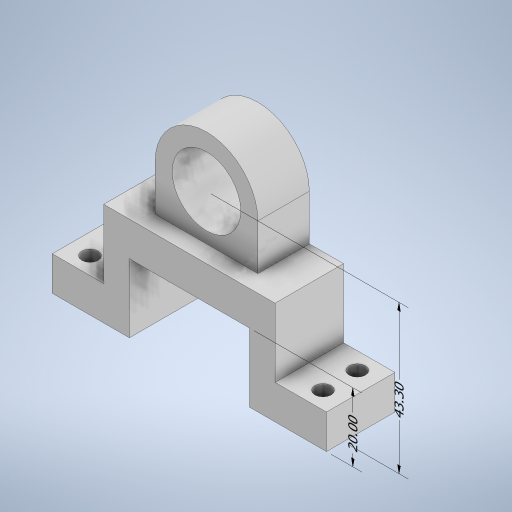
# Autodesk Inventor part: soporte_balineras
Saved by Autodesk Inventor 2023 (Build 270158000, 158)
## iProperties
Created: 2023-06-06
Part Number: soporte_balineras
Material: Genérico
Document SubType Name: Modeling
Designer: sergi
Density: 1 g/cm^3
Appearance: Valor por defecto
Author: sergi
Autodesk Inventor part; units mm, degrees
ref_plane "YZ Plane" through (0, 0, 0) normal (1, 0, 0) x (0, 1, 0)
ref_plane "XZ Plane" through (0, 0, 0) normal (0, 1, 0) x (-1, 0, 0)
ref_plane "XY Plane" through (0, 0, 0) normal (0, 0, 1) x (1, 0, 0)
sketch "Boceto1" plane through (0, 0, 0) normal (0, 0, 1) x (1, 0, 0)
  circle A0 centre (0, 23.4183) radius 10
  circle A1 centre (0, 23.4183) radius 15
  line L0 (-15, 23.4183) -> (-15, -2.7)
  line L1 (15, 23.4183) -> (15, -2.7)
  line L2 (-25, 0.1183) -> (25, 0.1183)
  line L3 (25, 0.1183) -> (25, 10.1183)
  line L4 (25, 10.1183) -> (-25, 10.1183)
  line L5 (-25, 10.1183) -> (-25, 0.1183)
  point P0 (0, 0)
  point P1 (0, 0.1183)
  point P2 (-15, 10.1183)
  point P3 (15, 10.1183)
  dimension "d0" = 20
  dimension "d1" = 30
  dimension "d2" = 50
  dimension "d11" = 10
  dimension "d23" = 23.3
  constraints: 12 end point, 2 centre point, 2 parallel, 2 point on circle, 2 vertical, 1 coincident, 1 horizontal, 1 midpoint, 1 perpendicular, 1 vertical alignment
  measures "d0" diameter of A0
  measures "d1" diameter of A1
  measures "d2" distance of L2.start L2.end
  measures "d11" distance of L2.end L3.end
  measures "d23" distance from line of L2 A0.centre
extrude "Extrusión1" add sketch "Boceto1" along normal blind 20 contours L4 L1 L2 L0 A1 | A1 L4 | L4 L3 L2 L1 | L0 L2 L5 L4 picked at (-1.1902, 9.6954)
extrude "Extrusión2" add sketch "Boceto1" along normal blind 15 contours A1 L4 | L1 L4 A1 | A1 L4 L0 picked at (0.4018, 11.2426)
sketch "Boceto3" plane through (-25, 0.1183, 0) normal (0, -1, 0) x (1, 0, 0)
  line L0 (0, 20) -> (50, 20) projected
  line L1 (7.5, 20) -> (42.5, 20)
  line L2 (42.5, 20) -> (42.5, 0)
  line L3 (42.5, 0) -> (7.5, 0)
  line L4 (7.5, 0) -> (7.5, 20)
  line L5 (0, 0) -> (50, 0) projected
  line L6 (0, 0) -> (50, 0) projected
  line L7 (50, 0) -> (50, 20) projected
  line L8 (0, 20) -> (50, 20) projected
  line L9 (0, 0) -> (0, 20) projected
  point P0 (25, 0)
  point P1 (25, 20)
  point P2 (25, 0)
  dimension "d8" = 35
  constraints: 8 end point, 2 midpoint, 2 parallel, 1 horizontal, 1 perpendicular, 1 point on line, 1 vertical alignment
  measures "d8" distance between parallel lines of L2 L4
extrude "Extrusión3" add sketch "Boceto3" along normal blind 20 contours L0 L4 L5 L9 | L0 L7 L5 L2
sketch "Boceto4" plane through (-25, 10.1183, 0) normal (-1, 0, 0) x (0, 0, 1)
  line L0 (0, -10.1183) -> (0, -30) projected
  line L1 (0, -30) -> (20, -30) projected
  line L2 (0, -20) -> (20, -20)
  line L3 (20, -20) -> (20, -30)
  line L4 (20, -30) -> (0, -30)
  line L5 (0, -30) -> (0, -20)
  dimension "d12" = 10
  constraints: 8 end point, 2 parallel, 1 horizontal, 1 perpendicular, 1 point on line
  measures "d12" distance between parallel lines of L1 L2
extrude "Extrusión4" add sketch "Boceto4" along normal blind 15
mirror "Simetría1" about plane through (0, 0, 0) normal (1, 0, 0) of "Extrusión4"
sketch "Boceto5" plane through (-25, -9.8817, 20) normal (0, 1, 0) x (1, 0, 0)
  circle A0 centre (-9, 15) radius 2.3813
  circle A1 centre (-9, 5) radius 2.3813
  line L0 (0, 20) -> (-15, 20) projected
  line L1 (0, 0) -> (-15, 0) projected
  line L2 (-15, 0) -> (-15, 20) projected
  point P0 (25, 20)
  dimension "d15" = 4.7625
  dimension "d16" = 4.7625
  dimension "d17" = 5
  dimension "d18" = 5
  dimension "d19" = 6
  dimension "d20" = 6
  constraints: 2 centre point
  measures "d15" diameter of A0
  measures "d16" diameter of A1
  measures "d17" distance from line of A0.centre L0
  measures "d18" distance from line of L1 A1.centre
  measures "d19" distance from line of L2 A1.centre
  measures "d20" distance from line of L2 A0.centre
extrude "Extrusión5" cut sketch "Boceto5" against normal through all
mirror "Simetría2" about plane through (0, 0, 0) normal (1, 0, 0) of "Extrusión5"
